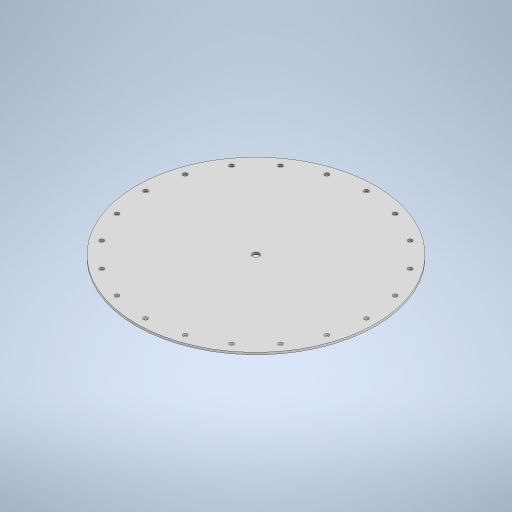
# Autodesk Inventor part: baseplate_azimuth_gear
Saved by Autodesk Inventor 2024 (Build 280153000, 153)
## iProperties
Created: 2025-12-10
Part Number: baseplate_azimuth_gear
Material: Generic
Document SubType Name: Modeling
Designer: schar
Density: 1 g/cm^3
Appearance: Default
Author: schar
Autodesk Inventor part; units mm, degrees
ref_plane "YZ Plane" through (0, 0, 0) normal (1, 0, 0) x (0, 1, 0)
ref_plane "XZ Plane" through (0, 0, 0) normal (0, 1, 0) x (-1, 0, 0)
ref_plane "XY Plane" through (0, 0, 0) normal (0, 0, 1) x (1, 0, 0)
sketch "Sketch1" plane through (0, 0, 0) normal (0, 1, 0) x (-1, 0, 0)
  circle A0 centre (0, 0) radius 110.292
  dimension "d0" = 220.584
  constraints: 1 centre point, 1 coincident
  measures "d0" diameter of A0
extrude "Extrusion1" add sketch "Sketch1" along normal blind 2
sketch "Sketch2" plane through (0, 2, 0) normal (0, 1, 0) x (1, 0, 0)
  line L0 (0, 0) -> (0, 101.796)
  circle A0 centre (0, 101.796) radius 2
  circle A1 centre (-31.4567, 96.8137) radius 2
  circle A2 centre (-59.8342, 82.3547) radius 2
  circle A3 centre (-82.3547, 59.8342) radius 2
  circle A4 centre (-96.8137, 31.4567) radius 2
  circle A5 centre (-101.796, 0) radius 2
  circle A6 centre (-96.8137, -31.4567) radius 2
  circle A7 centre (-82.3547, -59.8342) radius 2
  circle A8 centre (-59.8342, -82.3547) radius 2
  circle A9 centre (-31.4567, -96.8137) radius 2
  circle A10 centre (0, -101.796) radius 2
  circle A11 centre (31.4567, -96.8137) radius 2
  circle A12 centre (59.8342, -82.3547) radius 2
  circle A13 centre (82.3547, -59.8342) radius 2
  circle A14 centre (96.8137, -31.4567) radius 2
  circle A15 centre (101.796, 0) radius 2
  circle A16 centre (96.8137, 31.4567) radius 2
  circle A17 centre (82.3547, 59.8342) radius 2
  circle A18 centre (59.8342, 82.3547) radius 2
  circle A19 centre (31.4567, 96.8137) radius 2
  dimension "d3" = 101.796
  dimension "d4" = 4
  dimension "d7" = 360
  constraints: 20 centre point, 2 end point, 1 coincident, 1 vertical, 41 other
  measures "d3" distance of L0.start L0.end
  measures "d4" diameter of A0
hole "Hole1" at (-96.8137, 2, -31.4567) at (-82.3547, 2, -59.8342) at (-59.8342, 2, -82.3547) at (-31.4567, 2, -96.8137) at (31.4567, 2, -96.8137) at (59.8342, 2, -82.3547) at (82.3547, 2, -59.8342) at (96.8137, 2, -31.4567) at (101.796, 2, 0) at (96.8137, 2, 31.4567) at (82.3547, 2, 59.8342) at (59.8342, 2, 82.3547) at (31.4567, 2, 96.8137) at (0, 2, 101.796) at (-31.4567, 2, 96.8137) at (-59.8342, 2, 82.3547) at (-82.3547, 2, 59.8342) at (-96.8137, 2, 31.4567) at (-101.796, 2, 0) at (0, 2, -101.796) direction (0, -1, 0) diameter 4 end through all
sketch "Sketch4" plane through (0, 2, 0) normal (0, 1, 0) x (1, 0, 0)
  point P0 (0, 0)
  point P1 (0, 0)
  constraints: 1 coincident
hole "Hole2" at (0, 2, 0) direction (0, -1, 0) diameter 6 end through all
body "Solid1"
